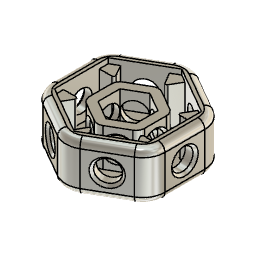
Core_PartA_x1 (Autodesk Fusion 360 design; units mm, degrees)
Autodesk Fusion 360 part; units mm, degrees
sketch "Sketch1" plane through (0, 0, 0) normal (0, 0, 1) x (1, 0, 0)
  line L0 (16.5, 9.5263) -> (0, 19.0526)
  line L1 (0, 19.0526) -> (-16.5, 9.5263)
  line L2 (-16.5, 9.5263) -> (-16.5, -9.5263)
  line L3 (-16.5, -9.5263) -> (0, -19.0526)
  line L4 (0, -19.0526) -> (16.5, -9.5263)
  line L5 (16.5, -9.5263) -> (16.5, 9.5263)
  dimension "d1" = 16.5
  measures "d1" distance of origin L5
extrude "Extrude1" add sketch "Sketch1" along normal blind 14
sketch "Sketch3" plane through (0, 0, 14) normal (0, 0, 1) x (-1, 0, 0)
  line L0 (-16.5, 9.5263) -> (-16.5, -9.5263)
  line L1 (-16.5, -9.5263) -> (0, -19.0526)
  line L2 (0, -19.0526) -> (16.5, -9.5263)
  line L3 (16.5, -9.5263) -> (16.5, 9.5263)
  line L4 (16.5, 9.5263) -> (0, 19.0526)
  line L5 (0, 19.0526) -> (-16.5, 9.5263)
  line L6 (-13.5, -7.7942) -> (0, -15.5885)
  line L7 (0, -15.5885) -> (13.5, -7.7942)
  line L8 (13.5, -7.7942) -> (13.5, 7.7942)
  line L9 (13.5, 7.7942) -> (0, 15.5885)
  line L10 (0, 15.5885) -> (-13.5, 7.7942)
  line L11 (-13.5, 7.7942) -> (-13.5, -7.7942)
  dimension "d7" = 13.5
  measures "d7" distance of origin L11
extrude "Extrude3" cut sketch "Sketch3" against normal blind 12.5 contours L6 L7 L8 L9 L10 L11
sketch "Sketch8" plane through (0, 0, 1.5) normal (0, 0, 1) x (-1, 0, 0)
  line L0 (-13.5, 7.7942) -> (-13.5, -7.7942)
  line L1 (-13.5, -7.7942) -> (0, -15.5885)
  line L2 (0, -15.5885) -> (13.5, -7.7942)
  line L3 (13.5, -7.7942) -> (13.5, 7.7942)
  line L4 (13.5, 7.7942) -> (0, 15.5885)
  line L5 (0, 15.5885) -> (-13.5, 7.7942)
  line L6 (-13.5, 7.7942) -> (-13.5, 5.1942)
  line L7 (-13.5, 7.7942) -> (-11.2483, 9.0942)
  line L8 (-11.2483, 9.0942) -> (-8.9967, 5.1942)
  line L9 (-8.9967, 5.1942) -> (-13.5, 5.1942)
  line L10 (-13.5, -7.7942) -> (-13.5, -5.1942)
  line L11 (-13.5, -7.7942) -> (-11.2483, -9.0942)
  line L12 (-11.2483, -9.0942) -> (-8.9967, -5.1942)
  line L13 (-8.9967, -5.1942) -> (-13.5, -5.1942)
  line L14 (13.5, 7.7942) -> (13.5, 5.1942)
  line L15 (13.5, 7.7942) -> (11.2483, 9.0942)
  line L16 (11.2483, 9.0942) -> (8.9967, 5.1942)
  line L17 (13.5, 5.1942) -> (8.9967, 5.1942)
  line L18 (0, 15.5885) -> (-2.2517, 14.2885)
  line L19 (0, 15.5885) -> (2.2517, 14.2885)
  line L20 (-2.2517, 14.2885) -> (0, 10.3885)
  line L21 (0, 10.3885) -> (2.2517, 14.2885)
  line L22 (13.5, -7.7942) -> (11.2483, -9.0942)
  line L23 (13.5, -7.7942) -> (13.5, -5.1942)
  line L24 (13.5, -5.1942) -> (8.9967, -5.1942)
  line L25 (11.2483, -9.0942) -> (8.9967, -5.1942)
  line L26 (0, -15.5885) -> (-2.2517, -14.2885)
  line L27 (0, -15.5885) -> (2.2517, -14.2885)
  line L28 (-2.2517, -14.2885) -> (0, -10.3885)
  line L29 (2.2517, -14.2885) -> (0, -10.3885)
  dimension "d19" = 2.6
  dimension "d20" = 2.6
  dimension "d23" = 2.6
  dimension "d24" = 2.6
  dimension "d25" = 2.6
  dimension "d26" = 2.6
  dimension "d27" = 2.6
  dimension "d28" = 2.6
  dimension "d29" = 2.6
  dimension "d30" = 2.6
  dimension "d31" = 2.6
  dimension "d32" = 2.6
  constraint coincident L0.start L5.end
  constraint parallel L0 L6
  constraint parallel L5 L7
  constraint perpendicular L7 L8
  constraint perpendicular L6 L9
  constraint coincident L0.end L1.start
  constraint parallel L0 L10
  constraint parallel L1 L11
  constraint perpendicular L11 L12
  constraint perpendicular L0 L13
  constraint coincident L3.end L4.start
  constraint parallel L3 L14
  constraint parallel L4 L15
  constraint perpendicular L4 L16
  constraint perpendicular L14 L17
  constraint coincident L4.end L5.start
  constraint parallel L5 L18
  constraint parallel L4 L19
  constraint perpendicular L5 L20
  constraint perpendicular L19 L21
  constraint coincident L2.end L3.start
  constraint parallel L2 L22
  constraint parallel L3 L23
  constraint perpendicular L23 L24
  constraint perpendicular L22 L25
  constraint coincident L1.end L2.start
  constraint parallel L1 L26
  constraint parallel L2 L27
  constraint perpendicular L26 L28
  constraint perpendicular L27 L29
  measures "d19" distance of L0.start L6.end
  measures "d20" distance of L0.start L7.end
  measures "d23" distance of L0.end L10.end
  measures "d24" distance of L0.end L11.end
  measures "d25" distance of L3.end L14.end
  measures "d26" distance of L3.end L15.end
  measures "d27" distance of L4.end L18.end
  measures "d28" distance of L4.end L19.end
  measures "d29" distance of L2.end L22.end
  measures "d30" distance of L2.end L23.end
  measures "d31" distance of L1.end L26.end
  measures "d32" distance of L1.end L27.end
extrude "Extrude7" add sketch "Sketch8" along normal blind 11 contours L0 L5 L6 L7 L8 L9 | L0 L1 L10 L11 L12 L13 | L4 L5 L18 L19 L20 L21 | L1 L2 L26 L27 L28 L29 | L3 L4 L14 L15 L16 L17 | L2 L3 L22 L23 L24 L25
fillet "Fillet1" radius 0.5 6 edges at (8.9967, -5.1942, 7) (8.9967, 5.1942, 7) (0, 10.3885, 7) (0, -10.3885, 7) (-8.9967, -5.1942, 7) (-8.9967, 5.1942, 7)
sketch "Sketch14" plane through (0, 0, 1.5) normal (0, 0, 1) x (-1, 0, 0)
  line L0 (-0.433, 11.1385) -> (-2.2517, 14.2885)
  line L1 (-2.2517, 14.2885) -> (-11.2483, 9.0942)
  line L2 (-11.2483, 9.0942) -> (-9.4297, 5.9442)
  arc A0 (-9.8627, 5.1942) -> (-9.4297, 5.9442) centre (-9.8627, 5.6942) ccw
  line L3 (-9.8627, 5.1942) -> (-13.5, 5.1942)
  line L4 (-13.5, 5.1942) -> (-13.5, -5.1942)
  line L5 (-13.5, -5.1942) -> (-9.8627, -5.1942)
  arc A1 (-9.4297, -5.9442) -> (-9.8627, -5.1942) centre (-9.8627, -5.6942) ccw
  line L6 (-9.4297, -5.9442) -> (-11.2483, -9.0942)
  line L7 (-11.2483, -9.0942) -> (-2.2517, -14.2885)
  line L8 (-2.2517, -14.2885) -> (-0.433, -11.1385)
  arc A2 (0.433, -11.1385) -> (-0.433, -11.1385) centre (0, -11.3885) ccw
  line L9 (0.433, -11.1385) -> (2.2517, -14.2885)
  line L10 (2.2517, -14.2885) -> (11.2483, -9.0942)
  line L11 (11.2483, -9.0942) -> (9.4297, -5.9442)
  arc A3 (9.8627, -5.1942) -> (9.4297, -5.9442) centre (9.8627, -5.6942) ccw
  line L12 (9.8627, -5.1942) -> (13.5, -5.1942)
  line L13 (13.5, -5.1942) -> (13.5, 5.1942)
  line L14 (13.5, 5.1942) -> (9.8627, 5.1942)
  arc A4 (9.4297, 5.9442) -> (9.8627, 5.1942) centre (9.8627, 5.6942) ccw
  line L15 (9.4297, 5.9442) -> (11.2483, 9.0942)
  line L16 (11.2483, 9.0942) -> (2.2517, 14.2885)
  line L17 (2.2517, 14.2885) -> (0.433, 11.1385)
  arc A5 (-0.433, 11.1385) -> (0.433, 11.1385) centre (0, 11.3885) ccw
  line L18 (-8, -4.6188) -> (0, -9.2376)
  line L19 (0, -9.2376) -> (8, -4.6188)
  line L20 (8, -4.6188) -> (8, 4.6188)
  line L21 (8, 4.6188) -> (0, 9.2376)
  line L22 (0, 9.2376) -> (-8, 4.6188)
  line L23 (-8, 4.6188) -> (-8, -4.6188)
extrude "Extrude12" add sketch "Sketch14" along normal blind 11 contours L18 L19 L20 L21 L22 L23
fillet "Fillet2" radius 2.5 6 edges at (8, -4.6188, 7) (8, 4.6188, 7) (0, -9.2376, 7) (-8, -4.6188, 7) (-8, 4.6188, 7) (0, 9.2376, 7)
sketch "Sketch15" plane through (0, 0, 12.5) normal (0, 0, 1) x (-1, 0, 0)
  arc A0 (-1.25, -8.5159) -> (1.25, -8.5159) centre (0, -6.3509) ccw
  line L0 (1.25, -8.5159) -> (6.75, -5.3405)
  arc A1 (6.75, -5.3405) -> (8, -3.1754) centre (5.5, -3.1754) ccw
  line L1 (8, -3.1754) -> (8, 3.1754)
  arc A2 (8, 3.1754) -> (6.75, 5.3405) centre (5.5, 3.1754) ccw
  line L2 (6.75, 5.3405) -> (1.25, 8.5159)
  arc A3 (1.25, 8.5159) -> (-1.25, 8.5159) centre (0, 6.3509) ccw
  line L3 (-1.25, 8.5159) -> (-6.75, 5.3405)
  arc A4 (-6.75, 5.3405) -> (-8, 3.1754) centre (-5.5, 3.1754) ccw
  line L4 (-8, 3.1754) -> (-8, -3.1754)
  arc A5 (-8, -3.1754) -> (-6.75, -5.3405) centre (-5.5, -3.1754) ccw
  line L5 (-6.75, -5.3405) -> (-1.25, -8.5159)
  line L6 (-5.5, -3.1754) -> (0, -6.3509)
  line L7 (0, -6.3509) -> (5.5, -3.1754)
  line L8 (5.5, -3.1754) -> (5.5, 3.1754)
  line L9 (5.5, 3.1754) -> (0, 6.3509)
  line L10 (0, 6.3509) -> (-5.5, 3.1754)
  line L11 (-5.5, 3.1754) -> (-5.5, -3.1754)
  dimension "d55" = 5.5
  measures "d55" distance of origin L11
extrude "Extrude13" cut sketch "Sketch15" against normal blind 10.5 contours L6 L7 L8 L9 L10 L11
sketch "Sketch16" plane through (0, 0, 2) normal (0, 0, 1) x (-1, 0, 0)
  line L0 (-5.5, 3.1754) -> (-5.5, -3.1754)
  line L1 (-5.5, -3.1754) -> (0, -6.3509)
  line L2 (0, -6.3509) -> (5.5, -3.1754)
  line L3 (5.5, -3.1754) -> (5.5, 3.1754)
  line L4 (5.5, 3.1754) -> (0, 6.3509)
  line L5 (0, 6.3509) -> (-5.5, 3.1754)
sketch "Sketch17" plane through (0, 0, 2) normal (0, 0, 1) x (-1, 0, 0)
  line L0 (-5.5, 3.1754) -> (-5.5, -3.1754)
  line L1 (-5.5, -3.1754) -> (0, -6.3509)
  line L2 (0, -6.3509) -> (5.5, -3.1754)
  line L3 (5.5, -3.1754) -> (5.5, 3.1754)
  line L4 (5.5, 3.1754) -> (0, 6.3509)
  line L5 (0, 6.3509) -> (-5.5, 3.1754)
  circle A0 centre (0, 0) radius 3.1
  dimension "d60" = 6.2
  constraint coincident A0.centre origin
  measures "d60" diameter of A0
extrude "Extrude15" cut sketch "Sketch17" against normal blind 4 contours A0
sketch "Sketch5" plane through (8.25, -14.2894, 0) normal (0.5, -0.866025, 0) x (0.866025, 0.5, 0)
  line L0 (-9.5263, 0) -> (9.5263, 0)
  line L1 (9.5263, 0) -> (9.5263, 14)
  line L2 (9.5263, 14) -> (-9.5263, 14)
  line L3 (-9.5263, 14) -> (-9.5263, 0)
  circle A0 centre (0, 7) radius 3.1
  dimension "d10" = 6.2
  measures "d10" diameter of A0
sketch "Sketch6" plane through (16.5, 0, 0) normal (1, 0, 0) x (0, 1, 0)
  line L0 (-9.5263, 0) -> (9.5263, 0)
  line L1 (9.5263, 0) -> (9.5263, 14)
  line L2 (9.5263, 14) -> (-9.5263, 14)
  line L3 (-9.5263, 14) -> (-9.5263, 0)
  circle A0 centre (0, 7) radius 3.1
  dimension "d13" = 6.2
  measures "d13" diameter of A0
sketch "Sketch7" plane through (8.25, 14.2894, 0) normal (0.5, 0.866025, 0) x (-0.866025, 0.5, 0)
  line L0 (-9.5263, 0) -> (9.5263, 0)
  line L1 (9.5263, 0) -> (9.5263, 14)
  line L2 (9.5263, 14) -> (-9.5263, 14)
  line L3 (-9.5263, 14) -> (-9.5263, 0)
  circle A0 centre (0, 7) radius 3.1
  dimension "d16" = 6.2
  measures "d16" diameter of A0
extrude "Extrude16" cut sketch "Sketch5" against normal blind 39 contours A0
extrude "Extrude17" cut sketch "Sketch6" against normal blind 41 contours A0
extrude "Extrude18" cut sketch "Sketch7" against normal blind 39 contours A0
fillet "Fillet3" radius 6.5 6 edges at (16.5, 9.5263, 7) (0, 19.0526, 7) (16.5, -9.5263, 7) (0, -19.0526, 7) (-16.5, -9.5263, 7) (-16.5, 9.5263, 7)
fillet "Fillet4" radius 2 24 edges at (-8.25, -14.2894, 0) (0, -18.047, 0) (8.25, -14.2894, 0) (15.6292, -9.0235, 0) (16.5, 0, 0) (15.6292, 9.0235, 0) (8.25, 14.2894, 0) (0, 18.047, 0) (-8.25, 14.2894, 0) (-15.6292, 9.0235, 0) (-16.5, 0, 0) (-15.6292, -9.0235, 0) (-15.6292, -9.0235, 14) (-8.25, -14.2894, 14) (0, -18.047, 14) (8.25, -14.2894, 14) (15.6292, -9.0235, 14) (16.5, 0, 14) (15.6292, 9.0235, 14) (8.25, 14.2894, 14) (0, 18.047, 14) (-8.25, 14.2894, 14) (-15.6292, 9.0235, 14) (-16.5, 0, 14)
chamfer "Chamfer1" distance 0.75 angle 45 13 edges at (10.753, 12.8443, 8.121) (-10.753, 12.8443, 5.879) (16.5, -2.8902, 8.121) (5.747, -15.7345, 8.121) (-5.747, -15.7345, 5.879) (-16.5, -2.8902, 5.879) (-8, -2.8902, 5.879) (-1.497, -8.3733, 5.879) (1.497, -8.3733, 8.121) (8, -2.8902, 8.121) (6.503, 5.4831, 8.121) (-6.503, 5.4831, 5.879) (2.8902, 1.121, 0)
